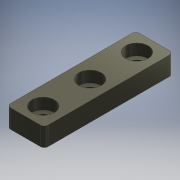
# Autodesk Inventor part: Belt Clamp
Saved by Autodesk Inventor 2016 (Build 200138000, 138)
## iProperties
Created: 2017-02-03
Part Number: Belt Clamp
Material: PC/ABS Plastic
Document SubType Name: Modeling
Designer: Scott
Density: 0.357273 g/cm^3
Appearance: Gunmetal
Author: Scott
## iProperties of the stored document Belt Clamp_3DPrint.ipt
Created: 2017-04-15
Part Number: Belt Clamp_3DPrint
Material: Generic
Document SubType Name: Modeling
Designer: Scott
Density: 1 g/cm^3
Appearance: Default
Author: Scott
Autodesk Inventor part; units mm, degrees
ref_plane "YZ Plane" through (0, 0, 0) normal (1, 0, 0) x (0, 1, 0)
ref_plane "XZ Plane" through (0, 0, 0) normal (0, 1, 0) x (-1, 0, 0)
ref_plane "XY Plane" through (0, 0, 0) normal (0, 0, 1) x (1, 0, 0)
sketch "Sketch1" plane through (0, 0, 0) normal (0, 0, 1) x (1, 0, 0)
  line L0 (0, 0) -> (10, 0)
  line L1 (10, 0) -> (10, 34.4)
  line L2 (10, 34.4) -> (0, 34.4)
  line L3 (0, 34.4) -> (0, 0)
  dimension "d0" = 34.4
  dimension "d1" = 10
  constraints: 8 end point, 2 parallel, 1 horizontal, 1 perpendicular
  measures "d0" distance of L0.end L1.end
  measures "d1" distance of L0.start L0.end
extrude "Extrusion1" add sketch "Sketch1" along normal blind 5
sketch "Sketch2" plane through (0, 0, 5) normal (0, 0, 1) x (1, 0, 0)
  line L0 (10, 34.4) -> (0, 34.4) projected
  line L1 (10, 0) -> (10, 34.4) projected
  line L2 (0, 34.4) -> (0, 0) projected
  line L3 (0, 0) -> (10, 0) projected
  line L4 (5, 34.4) -> (5, 0) construction
  line L5 (0, 17.2) -> (10, 17.2) construction
  point P0 (5, 29.7)
  point P1 (5, 4.7)
  point P2 (5, 17.2)
  dimension "d4" = 12.5
  dimension "d5" = 12.5
  constraints: 5 midpoint, 4 end point, 2 point on line
  measures "d4" distance from line of L5 point (5, 29.7)
  measures "d5" distance from line of point (5, 4.7) L5
hole "Hole1" at (5, 29.7, 5) at (5, 4.7, 5) at (5, 17.2, 5) direction (0, 0, -1) diameter 3.5 end through all counterbore diameter 6 counterbore depth 3
fillet "Fillet1" radius 1 4 edges at (0, 34.4, 2.5) (10, 34.4, 2.5) (10, 0, 2.5) (0, 0, 2.5)
equation "\"d5\" = d4"
body "Solid1"
